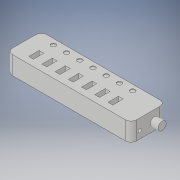
# Autodesk Inventor part: hub_dummy
Saved by Autodesk Inventor 2019 (Build 230136000, 136)
## iProperties
Created: 2019-04-16
Part Number: hub_dummy
Material: Generic
Document SubType Name: Modeling
Designer: zacha
Density: 1 g/cm^3
Appearance: Default
Author: zacha
Autodesk Inventor part; units mm, degrees
ref_plane "YZ Plane" through (0, 0, 0) normal (1, 0, 0) x (0, 1, 0)
ref_plane "XZ Plane" through (0, 0, 0) normal (0, 1, 0) x (-1, 0, 0)
ref_plane "XY Plane" through (0, 0, 0) normal (0, 0, 1) x (1, 0, 0)
sketch "Sketch1" plane through (0, 0, 0) normal (0, 1, 0) x (-1, 0, 0)
  line L0 (0, 0) -> (-160.5, 0)
  line L1 (-160.5, 0) -> (-160.5, 44.5)
  line L2 (-160.5, 44.5) -> (0, 44.5)
  line L3 (0, 44.5) -> (0, 0)
  dimension "d0" = 44.5
  dimension "d1" = 160.5
  constraints: 8 end point, 2 parallel, 1 horizontal, 1 perpendicular
  measures "d0" distance of L2.end L0.start
  measures "d1" distance of L0.start L0.end
extrude "Extrusion1" add sketch "Sketch1" along normal blind 23.6
fillet "Fillet1" radius 7.2 4 edges at (0, 11.8, 44.5) (160.5, 11.8, 44.5) (160.5, 11.8, 0) (0, 11.8, 0)
sketch "Sketch2" plane through (160.5, 0, 37.3) normal (1, 0, 0) x (0, 0, -1)
  circle A0 centre (4.15, 9.25) radius 2.25
  line L0 (-7.2, 23.6) -> (-7.2, 0) projected
  line L1 (6.4, 23.6) -> (6.4, 0) construction
  line L2 (0, 23.6) -> (30.1, 23.6) construction
  line L3 (30.1, 0) -> (0, 0) construction
  line L4 (13.7348, 11.5) -> (-5.9943, 11.5) construction
  line L5 (0, 0) -> (-7.2, 0) construction
  point P0 (37.3, 0)
  dimension "d5" = 4.5
  dimension "d7" = 13.6
  dimension "d8" = 11.5
  constraints: 4 end point, 2 point on line, 2 tangent, 1 centre point, 1 horizontal, 1 vertical
  measures "d5" diameter of A0
  measures "d7" distance between parallel lines of L0 L1
  measures "d8" distance between parallel lines of L5 L4
extrude "Extrusion2" cut sketch "Sketch2" against normal blind 10
sketch "Sketch3" plane through (160.5, 0, 37.3) normal (1, 0, 0) x (0, 0, -1)
  circle A0 centre (23, 10.3) radius 5.3
  line L0 (17.7, 15.6) -> (17.7, 1.2331) construction
  line L1 (17.7, 15.6) -> (23.008, 15.6) construction
  line L2 (30.1, 0) -> (0, 0) construction
  line L3 (37.3, 0) -> (37.3, 23.6) construction
  dimension "d11" = 10.6
  dimension "d12" = 15.6
  dimension "d13" = 19.6
  constraints: 4 end point, 2 tangent, 1 centre point, 1 horizontal, 1 vertical
  measures "d11" diameter of A0
  measures "d12" distance from line of L2 L1.end
  measures "d13" distance between parallel lines of L3 L0
extrude "Extrusion3" add sketch "Sketch3" along normal blind 10
sketch "Sketch4" plane through (0, 0, 7.2) normal (-1, 0, 0) x (0, 0, 1)
  line L0 (8.3, 14.15) -> (21.8, 14.15)
  line L1 (21.8, 14.15) -> (21.8, 7.35)
  line L2 (21.8, 7.35) -> (8.3, 7.35)
  line L3 (8.3, 7.35) -> (8.3, 14.15)
  line L4 (30.1, 0) -> (0, 0) projected
  line L5 (-7.2, 23.6) -> (-7.2, 0) projected
  line L6 (37.3, 0) -> (37.3, 23.6) projected
  dimension "d16" = 7.35
  dimension "d17" = 6.8
  dimension "d18" = 13.5
  dimension "d19" = 15.5
  dimension "d20" = 15.5
  constraints: 8 end point, 2 parallel, 1 horizontal, 1 perpendicular
  measures "d16" distance between parallel lines of L4 L2
  measures "d17" distance of L0.end L1.end
  measures "d18" distance of L0.start L0.end
  measures "d19" distance between parallel lines of L3 L5
  measures "d20" distance between parallel lines of L1 L6
extrude "Extrusion4" cut sketch "Sketch4" against normal blind 20
sketch "Sketch5" plane through (0, 23.6, 0) normal (0, 1, 0) x (1, 0, 0)
  line L0 (0.85, -43.7) -> (159.65, -43.7) construction
  line L1 (159.65, -43.7) -> (159.65, -0.8) construction
  line L2 (159.65, -0.8) -> (0.85, -0.8) construction
  line L3 (0.85, -0.8) -> (0.85, -43.7) construction
  line L4 (153.3, 0) -> (7.2, 0) construction
  line L5 (7.2, -44.5) -> (153.3, -44.5) construction
  line L6 (0, -7.2) -> (0, -37.3) construction
  line L7 (160.5, -37.3) -> (160.5, -7.2) construction
  line L8 (19.85, -36.15) -> (26.05, -36.15)
  line L9 (26.05, -36.15) -> (26.05, -22.65)
  line L10 (26.05, -22.65) -> (19.85, -22.65)
  line L11 (19.85, -22.65) -> (19.85, -36.15)
  line L12 (43.15, -36.15) -> (43.15, -22.65)
  line L13 (43.15, -22.65) -> (36.95, -22.65)
  line L14 (36.95, -22.65) -> (36.95, -36.15)
  line L15 (36.95, -36.15) -> (43.15, -36.15)
  line L16 (60.25, -36.15) -> (60.25, -22.65)
  line L17 (60.25, -22.65) -> (54.05, -22.65)
  line L18 (54.05, -22.65) -> (54.05, -36.15)
  line L19 (54.05, -36.15) -> (60.25, -36.15)
  line L20 (77.35, -36.15) -> (77.35, -22.65)
  line L21 (77.35, -22.65) -> (71.15, -22.65)
  line L22 (71.15, -22.65) -> (71.15, -36.15)
  line L23 (71.15, -36.15) -> (77.35, -36.15)
  line L24 (94.45, -36.15) -> (94.45, -22.65)
  line L25 (94.45, -22.65) -> (88.25, -22.65)
  line L26 (88.25, -22.65) -> (88.25, -36.15)
  line L27 (88.25, -36.15) -> (94.45, -36.15)
  line L28 (111.55, -36.15) -> (111.55, -22.65)
  line L29 (111.55, -22.65) -> (105.35, -22.65)
  line L30 (105.35, -22.65) -> (105.35, -36.15)
  line L31 (105.35, -36.15) -> (111.55, -36.15)
  line L32 (128.65, -36.15) -> (128.65, -22.65)
  line L33 (128.65, -22.65) -> (122.45, -22.65)
  line L34 (122.45, -22.65) -> (122.45, -36.15)
  line L35 (122.45, -36.15) -> (128.65, -36.15)
  point P0 (0, 0)
  dimension "d23" = 42.9
  dimension "d24" = 158.8
  dimension "d25" = 0.8
  dimension "d27" = 0.8
  dimension "d28" = 0.85
  dimension "d29" = 0.85
  dimension "d30" = 7.55
  dimension "d31" = 13.5
  dimension "d32" = 6.2
  dimension "d33" = 19
  dimension "d36" = 17.1
  constraints: 64 end point, 4 parallel, 3 horizontal, 2 perpendicular, 48 other
  measures "d23" distance of L0.end L1.end
  measures "d24" distance of L0.start L0.end
  measures "d25" distance between parallel lines of L2 L4
  measures "d27" distance between parallel lines of L0 L5
  measures "d28" distance between parallel lines of L3 L6
  measures "d29" distance between parallel lines of L1 L7
  measures "d30" distance between parallel lines of L0 L8
  measures "d31" distance of L8.end L9.end
  measures "d32" distance of L9.end L10.end
  measures "d33" distance between parallel lines of L11 L3
  measures "d36" distance of L9.end L12.end
extrude "Extrusion5" cut sketch "Sketch5" against normal blind 10
sketch "Sketch6" plane through (0, 23.6, 0) normal (0, 1, 0) x (1, 0, 0)
  circle A0 centre (22.95, -7.3) radius 3.1
  line L0 (19.85, -36.15) -> (19.85, -22.65) projected
  line L1 (26.05, -22.65) -> (26.05, -36.15) projected
  line L2 (153.3, 0) -> (7.2, 0) projected
  circle A1 centre (40.05, -7.3) radius 3.1
  circle A2 centre (57.15, -7.3) radius 3.1
  circle A3 centre (74.25, -7.3) radius 3.1
  circle A4 centre (91.35, -7.3) radius 3.1
  circle A5 centre (108.45, -7.3) radius 3.1
  circle A6 centre (125.55, -7.3) radius 3.1
  point P0 (0, 0)
  dimension "d43" = 4.2
  dimension "d46" = 17.1
  constraints: 7 centre point, 2 tangent, 1 horizontal, 12 other
  measures "d43" distance edge to line of A0 L2
  measures "d46" distance of A0.centre A1.centre
extrude "Extrusion6" cut sketch "Sketch6" against normal blind 1
equation "\"d20\" = d19"
equation "\"d27\" = d25"
equation "\"d29\" = d28"
body "Solid1"
